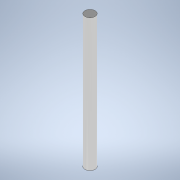
# Autodesk Inventor part: tija
Saved by Autodesk Inventor 2022 (Build 260153000, 153)
## iProperties
Created: 2022-03-04
Part Number: tija
Material: Steel, Alloy
Document SubType Name: Modeling
Designer: Oana
Density: 7.73 g/cm^3
Appearance: Chrome - Polished
Author: Oana
Autodesk Inventor part; units mm, degrees
ref_plane "YZ Plane" through (0, 0, 0) normal (1, 0, 0) x (0, 1, 0)
ref_plane "XZ Plane" through (0, 0, 0) normal (0, 1, 0) x (-1, 0, 0)
ref_plane "XY Plane" through (0, 0, 0) normal (0, 0, 1) x (1, 0, 0)
sketch "Sketch1" plane through (0, 0, 0) normal (0, 1, 0) x (-1, 0, 0)
  circle A0 centre (0, 0) radius 2.5
  dimension "d0" = 5
  constraints: 1 centre point, 1 coincident
  measures "d0" diameter of A0
extrude "Extrusion1" add sketch "Sketch1" along normal blind 65
equation "\"d0\" = diametru"
equation "\"d1\" = lungime"
equation "\"diametru\" = 5"
equation "\"lungime\" = 65"
body "Solid1"
